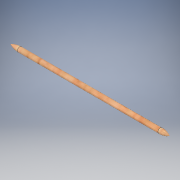
# Autodesk Inventor part: toothpick2
Saved by Autodesk Inventor 2016 (Build 200138000, 138)
## iProperties
Created: 2017-04-27
Part Number: toothpick2
Material: Generic
Document SubType Name: Modeling
Designer: wtse3759
Density: 1 g/cm^3
Appearance: Birch - Natural Polished
Author: wtse3759
Autodesk Inventor part; units mm, degrees
ref_plane "YZ Plane" through (0, 0, 0) normal (1, 0, 0) x (0, 1, 0)
ref_plane "XZ Plane" through (0, 0, 0) normal (0, 1, 0) x (-1, 0, 0)
ref_plane "XY Plane" through (0, 0, 0) normal (0, 0, 1) x (1, 0, 0)
sketch "Sketch1" plane through (0, 0, 0) normal (1, 0, 0) x (0, 1, 0)
  circle A0 centre (0, 0) radius 1.27
  dimension "d0" = 2.54
  constraints: 1 centre point, 1 coincident
  measures "d0" diameter of A0
extrude "Extrusion1" add sketch "Sketch1" along normal blind 76.2
sketch "Sketch2" plane through (0, 0, 0) normal (0, 1, 0) x (-1, 0, 0)
  line L0 (0, 0) -> (5.08, 0)
  line L1 (0, -1.27) -> (0, 1.27) projected
  line L2 (0, 0) -> (0, -1.27)
  line L3 (-76.2, 1.27) -> (-76.2, -1.27) projected
  line L4 (-76.2, 0) -> (-81.28, 0)
  line L5 (-76.2, 0) -> (-76.2, -1.27)
  arc A0 (0, -1.27) -> (5.08, 0) centre (-0.0427, 9.6958) ccw
  arc A1 (-81.28, 0) -> (-76.2, -1.27) centre (-76.9847, 6.3863) ccw
  line L6 (14.8466, 0) -> (-52.981, 0) projected
  dimension "d3" = 5.08
  dimension "d4" = 5.08
  constraints: 8 end point, 4 point on circle, 2 centre point, 2 collinear, 2 horizontal, 1 midpoint
  measures "d3" distance of L0.start L0.end
  measures "d4" distance of L4.start L4.end
revolve "Revolution1" add sketch "Sketch2" angle 360 about axis through (-10, 0, 0) along (1, 0, 0)
body "Solid1"
